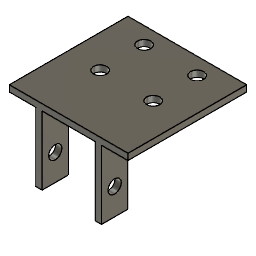
Gantry Sliding Brackets (Autodesk Fusion 360 design; units mm, degrees)
part number: 2026-04-23-21-07-36-866
Autodesk Fusion 360 part; units mm, degrees
sketch "Sketch1" plane through (0, 0, 0) normal (0, 0, 1) x (1, 0, 0)
  line L0 (-13.45, 12) -> (31.55, 12)
  line L1 (31.55, 12) -> (31.55, -33)
  line L2 (31.55, -33) -> (-13.45, -33)
  line L3 (-13.45, -33) -> (-13.45, 12)
  line L4 (-3.4, -33) -> (-1, -33)
  line L5 (-1, -33) -> (-1, -23)
  line L6 (-1, -23) -> (-3.4, -23)
  line L7 (-3.4, -23) -> (-3.4, -33)
  line L8 (19.1, -23) -> (19.1, -33)
  line L9 (21.5, -23) -> (19.1, -23)
  line L10 (21.5, -33) -> (21.5, -23)
  line L11 (19.1, -33) -> (21.5, -33)
  circle A0 centre (-1, 5.65) radius 2.5
  circle A1 centre (-1, 5.65) radius 7.65
  circle A2 centre (19.1, 5.65) radius 7.65
  circle A3 centre (19.1, 5.65) radius 2.5
  circle A4 centre (-1, -11) radius 2.5
  circle A5 centre (19.1, -11) radius 2.5
  circle A6 centre (-1, -11) radius 9
  circle A7 centre (19.1, -11) radius 9
  dimension "d1" = 45
  dimension "d2" = 45
  dimension "d3" = 10
  dimension "d4" = 2.4
  dimension "d5" = 10.05
  dimension "d7" = 2.4
  dimension "d8" = 20.1
  dimension "d9" = 5
  dimension "d10" = 6.35
  dimension "d11" = 15.3
  dimension "d13" = 5
  dimension "d14" = 15.3
  dimension "d15" = 20.1
  dimension "d16" = 12.45
  dimension "d25" = 5
  dimension "d26" = 5
  dimension "d27" = 20.1
  dimension "d28" = 12.45
  dimension "d31" = 18
  dimension "d32" = 18
  constraint horizontal L0
  constraint vertical L1
  constraint horizontal L2
  constraint vertical L3
  constraint horizontal L4
  constraint vertical L5
  constraint horizontal L6
  constraint vertical L7
  constraint coincident L2 L4.start
  constraint horizontal L11
  constraint vertical L10
  constraint horizontal L9
  constraint vertical L8
  constraint concentric A0 A1
  constraint concentric A2 A3
  constraint concentric A4 A6
  constraint concentric A5 A7
  measures "d1" distance of L0.start L2.end
  measures "d2" distance of L1 L3
  measures "d3" distance of L4.start L6.end
  measures "d4" distance of L5 L7
  measures "d5" distance of L3 L7
  measures "d7" distance of L8 L10
  measures "d8" distance of L5 L8
  measures "d9" diameter of A0
  measures "d10" distance of L0 A0.centre
  measures "d11" diameter of A1
  measures "d13" diameter of A3
  measures "d14" diameter of A2
  measures "d15" distance of A0.centre A2.centre
  measures "d16" distance of L1 A2.centre
  measures "d25" diameter of A4
  measures "d26" diameter of A5
  measures "d27" distance of A4.centre A5.centre
  measures "d28" distance of L1 A5.centre
  measures "d31" diameter of A6
  measures "d32" diameter of A7
extrude "Extrude1" add sketch "Sketch1" along normal blind 2.4 contours A7 | A6 | L0 L1 L2 L3 L5 L6 L7 L8 L9 L10 A1 A2 | L0 A1 | L2 L4 L5 L6 L7 | L0 A2 | L2 L8 L9 L10 L11 | A4 | A5 picked at (-1.0623, 10.7143) picked at (19.0377, 10.7143)
extrude "Extrude2" add sketch "Sketch1" against normal blind 26 contours L2 L4 L5 L6 L7 | L2 L8 L9 L10 L11
sketch "Sketch2" plane through (21.5, 0, 0) normal (1, 0, 0) x (0, 1, 0)
  line L0 (-23, 0) -> (-33, 0)
  line L1 (-33, 0) -> (-33, -26)
  line L2 (-33, -26) -> (-23, -26)
  line L3 (-23, -26) -> (-23, 0)
  circle A0 centre (-28, -16) radius 2.5
  dimension "d21" = 5
  dimension "d22" = 10
  measures "d21" diameter of A0
  measures "d22" distance of L2 A0.centre
extrude "Extrude3" cut sketch "Sketch2" against normal blind 30 contours A0
extrude "Extrude4" cut sketch "Sketch1" along normal blind 3 contours A4 | A5
